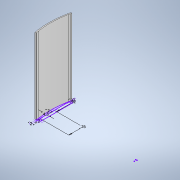
# Autodesk Inventor part: face_v2
Saved by Autodesk Inventor 2022 (Build 260153000, 153)
## iProperties
Created: 2023-03-27
Part Number: face_v2
Material: Generic
Document SubType Name: Modeling
Designer: emp
Density: 1 g/cm^3
Appearance: Default
Author: emp
Autodesk Inventor part; units mm, degrees
ref_plane "YZ Plane" through (0, 0, 0) normal (1, 0, 0) x (0, 1, 0)
ref_plane "XZ Plane" through (0, 0, 0) normal (0, 1, 0) x (-1, 0, 0)
ref_plane "XY Plane" through (0, 0, 0) normal (0, 0, 1) x (1, 0, 0)
sketch "Sketch1" plane through (0, 0, 0) normal (0, 1, 0) x (-1, 0, 0)
  line L0 (0.0938, -37.5) -> (4.5938, -37.5) construction
  line L1 (0, 0) -> (2, 0) construction
  line L2 (4.5938, -37.5) -> (6.5938, -37.5) construction
  line L3 (0, -75) -> (2, -75) construction
  arc A0 (2.4733, -73) -> (4.082, -8.9832) centre (-151.9057, -37.0919) ccw
  line L4 (2.0086, -8.9832) -> (4.082, -8.9832)
  line L5 (0, -73) -> (2.4733, -73)
  arc A1 (2.3337, -10.8228) -> (2.0086, -8.9832) centre (-154, -37.5) ccw
  arc A2 (0.4733, -73) -> (0.9193, -71) centre (-154, -37.5) ccw
  arc A3 (1.7305, -67.5) -> (2.9896, -15) centre (-154, -37.5) ccw
  line L6 (1.3383, -67.5) -> (1.3383, -5.3327) construction
  line L7 (2.9896, -15) -> (1.3383, -15) construction
  line L8 (1.3383, -15) -> (1.3383, -13)
  arc A4 (2.9896, -15) -> (2.3337, -10.8228) centre (-153.9981, -37.5133) ccw
  line L9 (1.3383, -13) -> (2.6898, -13)
  arc A5 (0.9193, -71) -> (1.7305, -67.5) centre (-153.0722, -33.465) ccw
  line L10 (1.3383, -15) -> (1.3383, -68.25)
  line L11 (2.9896, -15) -> (5.0472, -15)
  line L12 (1.8227, -67.0175) -> (3.7437, -67.0175)
  line L13 (-3.6617, -10.8228) -> (-3.6617, -71)
  line L14 (2.3337, -10.8228) -> (-3.6617, -10.8228)
  line L15 (1.3383, -13.5728) -> (-3.6617, -13.5728)
  line L16 (1.5637, -68.25) -> (-3.6617, -68.25)
  line L17 (0.9193, -71) -> (-3.6617, -71)
  point P0 (0, -7)
  point P1 (2, 0)
  point P2 (0, -9)
  point P3 (0, -41)
  point P4 (0, -15)
  point P5 (0, -67.5)
  point P6 (0, -69)
  point P7 (0, -13)
  point P8 (2.595, -13)
  dimension "d15" = 4.5
  dimension "d17" = 2
  dimension "d18" = 2
  dimension "d19" = 2
  dimension "d20" = 2
  dimension "d21" = 2
  dimension "d22" = 32
  dimension "d24" = 26
  constraints: 36 end point, 20 point on circle, 8 horizontal, 6 centre point, 6 coincident, 5 point on line, 3 perpendicular, 2 collinear, 2 parallel, 1 equal radius, 1 vertical
  measures "d15" distance of L0.start L0.end
  measures "d17" distance of L1.start L1.end
  measures "d18" distance of L0.end L2.end
  measures "d19" distance of L3.start L3.end
  measures "d20" distance of point (0, -75) L5.start
  measures "d21" distance of point (0, -9) point (0, -7)
  measures "d22" distance of L5.start point (0, -41)
  measures "d24" distance of point (0, -41) point (0, -15)
extrude "Extrusion1" add sketch "Sketch1" along normal blind 138 contours L5 A2 A5 A3 L12 A0 | L12 A3 L11 A0 | L11 A4 A1 L4 A0
body "Solid1"
